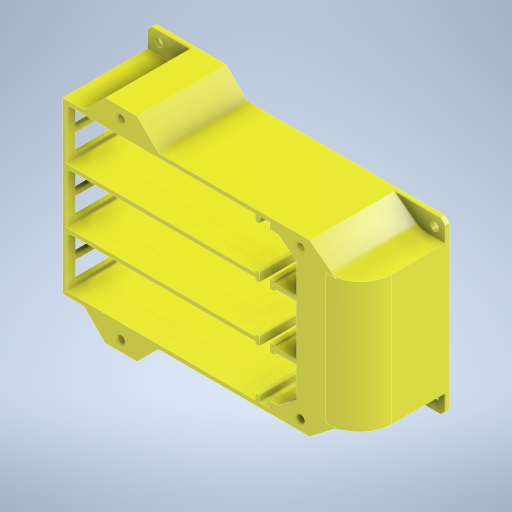
# Autodesk Inventor part: MainBody
Saved by Autodesk Inventor 2024.2 (Build 282272000, 272)
## iProperties
Created: 2024-05-26
Part Number: MainBody
Material: PBT Plastic
Document SubType Name: Modeling
Designer: simon
Density: 1.31 g/cm^3
Appearance: Yellow
Author: simon
Autodesk Inventor part; units mm, degrees
ref_plane "YZ Plane" through (0, 0, 0) normal (1, 0, 0) x (0, 1, 0)
ref_plane "XZ Plane" through (0, 0, 0) normal (0, 1, 0) x (-1, 0, 0)
ref_plane "XY Plane" through (0, 0, 0) normal (0, 0, 1) x (1, 0, 0)
sketch "Sketch1" plane through (0, 0, 0) normal (0, 0, 1) x (1, 0, 0)
  line L0 (0, 0) -> (140, 0)
  line L1 (140, 0) -> (140, 80)
  line L2 (140, 80) -> (0, 80)
  line L3 (0, 80) -> (0, 0)
  line L4 (109.9, 68.55) -> (138, 68.55)
  line L5 (138, 68.55) -> (138, 11.45)
  line L6 (138, 11.45) -> (109.9, 11.45)
  line L7 (109.9, 11.45) -> (109.9, 68.55)
  dimension "d0" = 140
  dimension "d1" = 80
  dimension "d2" = 28.1
  dimension "d3" = 57.1
  dimension "d4" = 11.45
  dimension "d5" = 2
  constraints: 16 end point, 4 parallel, 2 horizontal, 2 perpendicular
  measures "d0" distance of L2.end L1.end
  measures "d1" distance of L1.end L0.end
  measures "d2" distance of L5.end L6.end
  measures "d3" distance of L4.end L5.end
  measures "d4" distance between parallel lines of L2 L4
  measures "d5" distance between parallel lines of L1 L5
extrude "Extrusion1" add sketch "Sketch1" against normal blind 2
sketch "Sketch2" plane through (0, 0, 0) normal (0, 0, 1) x (1, 0, 0)
  line L0 (109.9, 68.55) -> (109.9, 11.45) projected
  line L1 (109.9, 68.55) -> (94.9, 80)
  line L2 (0, 80) -> (140, 80) projected
  line L3 (138, 68.55) -> (109.9, 68.55) projected
  line L4 (109.9, 68.55) -> (113.1962, 68.55)
  line L5 (113.1962, 68.55) -> (98.1962, 80)
  line L6 (98.1962, 80) -> (94.9, 80)
  line L7 (109.9, 11.45) -> (138, 11.45) projected
  line L8 (109.9, 11.45) -> (94.9, 0)
  line L9 (140, 0) -> (0, 0) projected
  line L10 (98.1962, 0) -> (113.1962, 11.45)
  line L11 (113.1962, 11.45) -> (109.9, 11.45)
  line L12 (94.9, 0) -> (98.1962, 0)
  point P0 (113.1962, 11.45)
  point P1 (135, 80)
  point P2 (135, 0)
  dimension "d8" = 2
  dimension "d9" = 15
  dimension "d10" = 2
  dimension "d11" = 15
  constraints: 16 end point, 4 point on line, 3 parallel, 1 collinear, 1 perpendicular
  measures "d8" distance between parallel lines of L5 L1
  measures "d9" horizontal distance of L1.end L0.start
  measures "d10" distance between parallel lines of L10 L8
  measures "d11" horizontal distance of L8.end L0.end
extrude "Extrusion2" add sketch "Sketch2" along normal blind 40
sketch "Sketch3" plane through (109.9, 68.55, -2) normal (0, -1, 0) x (1, 0, 0)
  line L0 (3.2962, 2) -> (28.1, 2) projected
  line L1 (28.1, 2) -> (30.1, 2)
  line L2 (30.1, 2) -> (30.1, 27)
  line L3 (30.1, 27) -> (28.1, 27)
  line L4 (28.1, 27) -> (28.1, 2)
  line L5 (-15, 42) -> (0, 42) projected
  line L6 (0, 42) -> (14, 42)
  line L7 (14, 42) -> (14, 40)
  line L8 (14, 40) -> (0, 40)
  line L9 (0, 40) -> (0, 42)
  arc A0 (30.1, 27) -> (14, 42) centre (15.1001, 27.0404) ccw
  arc A1 (28.1, 27) -> (14, 40) centre (14.1357, 26.0007) ccw
  point P0 (-109.9, 2)
  dimension "d14" = 2
  dimension "d15" = 25
  dimension "d16" = 14
  dimension "d17" = 2
  dimension "d18" = 15
  dimension "d19" = 14
  constraints: 16 end point, 4 parallel, 4 point on circle, 2 centre point, 2 horizontal, 2 perpendicular
  measures "d14" distance of L3.end L2.end
  measures "d15" distance of L1.end L2.end
  measures "d16" distance of L7.end L8.end
  measures "d17" distance of L6.end L7.end
  measures "d18" radius of A0
  measures "d19" radius of A1
extrude "Extrusion3" add sketch "Sketch3" along normal blind 59.1 and the other way blind 2
sketch "Sketch4" plane through (109.9, 9.45, -2) normal (0, -1, 0) x (1, 0, 0)
  line L0 (0.6761, 42) -> (0.6761, 40) projected
  line L1 (0.6761, 42) -> (0.6761, 2)
  line L2 (30.1, 2) -> (-11.7038, 2) projected
  line L3 (30.1, 2) -> (30.1, 0) projected
  line L4 (0.6761, 2) -> (30.1, 2)
  line L5 (30.1, 27) -> (30.1, 2) projected
  line L6 (30.1, 2) -> (30.1, 27)
  line L7 (14, 42) -> (0.6761, 42) projected
  line L8 (0.6761, 42) -> (14, 42)
  arc A0 (30.1, 27) -> (14, 42) centre (15.1001, 27.0404) ccw projected
  arc A1 (30.1, 27) -> (14, 42) centre (15.1001, 27.0404) ccw
  point P0 (-109.9, 2)
  point P1 (0.6761, 40)
  point P2 (25.1, 2)
  point P3 (25.1, 2)
  constraints: 8 end point, 2 collinear, 2 point on circle, 1 centre point, 1 concentric, 1 perpendicular, 1 point on line, 1 vertical
extrude "Extrusion4" add sketch "Sketch4" against normal blind 2
sketch "Sketch5" plane through (109.9, 70.55, -2) normal (0, 1, 0) x (1, 0, 0)
  line L0 (14, -42) -> (0.6761, -42) projected
  line L1 (0.6761, -2) -> (0.6761, -42) projected
  line L2 (0.6761, -42) -> (0.6761, -2)
  line L3 (30.1, -2) -> (0.6761, -2) projected
  line L4 (0.6761, -2) -> (30.1, -2)
  line L5 (30.1, -27) -> (30.1, -2) projected
  line L6 (30.1, -2) -> (30.1, -27)
  line L7 (0.6761, -42) -> (14, -42)
  arc A0 (14, -42) -> (30.1, -27) centre (15.1001, -27.0404) ccw
  point P0 (-109.9, -2)
  constraints: 8 end point, 3 collinear, 2 point on circle, 1 centre point, 1 perpendicular
extrude "Extrusion5" add sketch "Sketch5" against normal blind 2
sketch "Sketch6" plane through (0, 0, 0) normal (0, 0, 1) x (1, 0, 0)
  line L0 (110.5761, 70.55) -> (98.1962, 80) projected
  line L1 (0, 0) -> (98.1962, 0)
  line L2 (98.1962, 0) -> (98.1962, 80)
  line L3 (98.1962, 80) -> (0, 80)
  line L4 (0, 80) -> (0, 0)
  line L5 (2, 2) -> (96.1962, 2)
  line L6 (96.1962, 2) -> (96.1962, 78)
  line L7 (96.1962, 78) -> (2, 78)
  line L8 (2, 78) -> (2, 2)
  line L9 (96.1962, 78) -> (98.1962, 78)
  line L10 (96.1962, 2) -> (98.1962, 2)
  dimension "d34" = 2
  dimension "d35" = 2
  dimension "d36" = 2
  dimension "d37" = 2
  constraints: 20 end point, 4 parallel, 4 perpendicular, 2 horizontal, 2 point on line
  measures "d34" distance between parallel lines of L8 L4
  measures "d35" distance between parallel lines of L5 L1
  measures "d36" distance between parallel lines of L3 L7
  measures "d37" distance between parallel lines of L6 L2
extrude "Extrusion6" add sketch "Sketch6" along normal blind 40 contours L4 L3 L2 L9 L7 L8 L5 L10 L1
sketch "Sketch7" plane through (0, 0, 0) normal (0, 0, 1) x (1, 0, 0)
  line L0 (-10, 53) -> (150, 53) construction
  line L1 (-7.9797, 27) -> (152.0203, 27) construction
  line L2 (0, 80) -> (0, 0) construction
  line L3 (2, 78) -> (97.5201, 78) construction
  line L4 (97.5201, 2) -> (2, 2) construction
  line L5 (2, 2) -> (2, 78) projected
  line L6 (2, 54) -> (92.52, 54)
  line L7 (92.52, 54) -> (92.52, 52)
  line L8 (92.52, 52) -> (2, 52)
  line L9 (2, 52) -> (2, 54)
  line L10 (2, 28) -> (92.52, 28)
  line L11 (92.52, 28) -> (92.52, 26)
  line L12 (92.52, 26) -> (2, 26)
  line L13 (2, 26) -> (2, 28)
  line L14 (0, 80) -> (140, 80) projected
  line L15 (90.5201, 80) -> (92.5201, 80)
  line L16 (92.5201, 80) -> (92.5201, 75)
  line L17 (92.5201, 75) -> (90.5201, 75)
  line L18 (90.5201, 75) -> (90.5201, 80)
  line L19 (97.5201, 78) -> (2, 78) projected
  line L20 (97.5201, 78) -> (97.5201, 75)
  line L21 (97.5201, 75) -> (101.4502, 75)
  line L22 (109.9, 68.55) -> (97.5201, 78) projected
  line L23 (101.4502, 75) -> (97.5201, 78)
  line L24 (97.5201, 78) -> (97.5201, 78)
  line L25 (97.5201, 2) -> (109.9, 11.45) projected
  line L26 (92.5201, 2) -> (90.5201, 2)
  line L27 (90.5201, 2) -> (90.5201, 5)
  line L28 (90.5201, 5) -> (92.5201, 5)
  line L29 (92.5201, 5) -> (92.5201, 2)
  line L30 (92.5201, 55) -> (90.5201, 55)
  line L31 (90.5201, 55) -> (90.5201, 51)
  line L32 (90.5201, 51) -> (92.5201, 51)
  line L33 (92.5201, 51) -> (92.5201, 55)
  line L34 (92.5201, 29) -> (90.52, 29)
  line L35 (90.52, 29) -> (90.52, 25)
  line L36 (90.52, 25) -> (92.5201, 25)
  line L37 (92.5201, 25) -> (92.5201, 29)
  line L38 (97.5201, 55) -> (99.5201, 55)
  line L39 (99.5201, 55) -> (99.5201, 51)
  line L40 (99.5201, 51) -> (97.5201, 51)
  line L41 (97.5201, 51) -> (97.5201, 55)
  line L42 (97.5201, 29) -> (99.5201, 29)
  line L43 (99.5201, 29) -> (99.5201, 25)
  line L44 (99.5201, 25) -> (97.5201, 25)
  line L45 (97.5201, 25) -> (97.5201, 29)
  line L46 (109.9, 68.55) -> (109.9, 11.45) projected
  line L47 (97.5201, 54) -> (109.9, 54)
  line L48 (109.9, 54) -> (109.9, 52)
  line L49 (109.9, 52) -> (97.5201, 52)
  line L50 (97.5201, 52) -> (97.5201, 54)
  line L51 (109.9, 28) -> (97.5201, 28)
  line L52 (97.5201, 28) -> (97.5201, 26)
  line L53 (97.5201, 26) -> (109.9, 26)
  line L54 (109.9, 26) -> (109.9, 28)
  line L55 (97.5201, 2) -> (97.5201, 5)
  line L56 (97.5201, 5) -> (101.4502, 5)
  line L57 (97.5201, 2) -> (101.4502, 5)
  line L58 (0, 0) -> (98.1962, 0) projected
  point P0 (135, 80)
  point P1 (102.7603, 6)
  point P2 (92.5201, 3.5)
  point P3 (91.5201, 55)
  point P4 (90.52, 26)
  point P5 (90.52, 28)
  point P6 (2, 26)
  point P7 (90.5201, 54)
  point P8 (2, 52)
  point P9 (90.5201, 52)
  point P10 (99.5201, 26)
  point P11 (99.5201, 28)
  point P12 (99.5201, 52)
  point P13 (99.5201, 54)
  dimension "d40" = 160
  dimension "d41" = 10
  dimension "d44" = 90.52
  dimension "d45" = 1
  dimension "d46" = 2
  dimension "d47" = 1
  dimension "d48" = 2
  dimension "d49" = 2
  dimension "d54" = 5
  dimension "d55" = 3
  dimension "d56" = 5
  dimension "d57" = 3
  dimension "d60" = 2
  dimension "d61" = 3
  dimension "d62" = 2
  dimension "d63" = 4
  dimension "d64" = 2
  dimension "d65" = 1.9999
  dimension "d66" = 4
  dimension "d67" = 2
  dimension "d68" = 2
  dimension "d69" = 2.0001
  dimension "d70" = 2
  dimension "d71" = 5
  dimension "d72" = 4
  dimension "d73" = 2
  dimension "d74" = 4
  dimension "d75" = 5
  dimension "d78" = 2
  dimension "d79" = 2
  dimension "d80" = 3
  dimension "d81" = 5
  dimension "d105" = 27
  dimension "d106" = 27
  constraints: 98 end point, 20 parallel, 14 perpendicular, 13 point on line, 12 horizontal, 5 collinear, 2 midpoint, 1 vertical
  measures "d40" distance of L0.start L0.end
  measures "d41" distance from line of L0.start L2
  measures "d44" distance of L7.end L8.end
  measures "d45" distance between parallel lines of L6 L0
  measures "d46" distance of L6.end L7.end
  measures "d47" distance between parallel lines of L10 L1
  measures "d48" distance of L10.end L11.end
  measures "d49" distance of L16.end L17.end
  measures "d54" distance between parallel lines of L16 L20
  measures "d55" distance between parallel lines of L3 L21
  measures "d56" distance from line of L3.end L16
  measures "d57" distance between parallel lines of L3 L17
  measures "d60" distance of L27.end L28.end
  measures "d61" distance from line of L26.end L28
  measures "d62" distance of L30.start L30.end
  measures "d63" distance of L32.end L30.start
  measures "d64" distance from line of L0 point (91.52, 55)
  measures "d65" distance from line of L7.end L31
  measures "d66" distance of L36.end L34.start
  measures "d67" distance between parallel lines of L1 L36
  measures "d68" distance from line of L10.end L35
  measures "d69" distance between parallel lines of L37 L35
  measures "d70" distance of L38.start L38.end
  measures "d71" distance between parallel lines of L33 L41
  measures "d72" distance of L38.end L39.end
  measures "d73" distance of L42.start L42.end
  measures "d74" distance of L42.end L43.end
  measures "d75" distance between parallel lines of L37 L45
  measures "d78" distance between parallel lines of L49 L47
  measures "d79" distance of L53.end L51.start
  measures "d80" distance of L4.start L55.end
  measures "d81" distance between parallel lines of L29 L55
  measures "d105" distance between parallel lines of L0 L14
  measures "d106" distance between parallel lines of L1 L58
extrude "Extrusion7" add sketch "Sketch7" along normal blind 40
sketch "Sketch8" plane through (0, 0, -2) normal (-1, 0, 0) x (0, 0, 1)
  line L0 (-10, 66) -> (50, 66) construction
  line L1 (-9.3981, 40) -> (50.6019, 40) construction
  line L2 (-9.3981, 14) -> (50.6019, 14) construction
  line L3 (0, 0) -> (0, 80) construction
  line L4 (0, 80) -> (42, 80) construction
  line L5 (4, 76) -> (38, 76)
  line L6 (38, 76) -> (38, 56)
  line L7 (38, 56) -> (4, 56)
  line L8 (4, 56) -> (4, 76)
  line L9 (42, 0) -> (0, 0) projected
  line L10 (4, 50) -> (38, 50)
  line L11 (38, 50) -> (38, 30)
  line L12 (38, 30) -> (4, 30)
  line L13 (4, 30) -> (4, 50)
  line L14 (4, 24) -> (38, 24)
  line L15 (38, 24) -> (38, 4)
  line L16 (38, 4) -> (4, 4)
  line L17 (4, 4) -> (4, 24)
  line L18 (42, 80) -> (42, 0) projected
  line L19 (38, 67) -> (4, 67)
  line L20 (4, 67) -> (4, 65)
  line L21 (4, 65) -> (38, 65)
  line L22 (38, 65) -> (38, 67)
  line L23 (38, 41) -> (4, 41)
  line L24 (4, 41) -> (4, 39)
  line L25 (4, 39) -> (38, 39)
  line L26 (38, 39) -> (38, 41)
  line L27 (38, 15) -> (4, 15)
  line L28 (4, 15) -> (4, 13)
  line L29 (4, 13) -> (38, 13)
  line L30 (38, 13) -> (38, 15)
  point P0 (2, 0)
  point P1 (4, 15)
  point P2 (38, 39)
  point P3 (4, 41)
  point P4 (4, 67)
  dimension "d82" = 60
  dimension "d83" = 10
  dimension "d87" = 20
  dimension "d88" = 10
  dimension "d89" = 34
  dimension "d90" = 4
  dimension "d91" = 40
  dimension "d93" = 34
  dimension "d94" = 20
  dimension "d95" = 4
  dimension "d96" = 10
  dimension "d97" = 20
  dimension "d98" = 10
  dimension "d99" = 34
  dimension "d100" = 4
  dimension "d103" = 26
  dimension "d104" = 26
  dimension "d107" = 2
  dimension "d108" = 1
  dimension "d109" = 2
  dimension "d110" = 1
  dimension "d111" = 2
  dimension "d112" = 1
  constraints: 54 end point, 12 parallel, 9 horizontal, 6 perpendicular, 6 point on line
  measures "d82" distance of L0.start L0.end
  measures "d83" distance from line of L3 L0.start
  measures "d87" distance of L5.end L6.end
  measures "d88" distance between parallel lines of L0 L7
  measures "d89" distance between parallel lines of L6 L8
  measures "d90" distance between parallel lines of L3 L8
  measures "d91" distance between parallel lines of L1 L4
  measures "d93" distance of L10.start L10.end
  measures "d94" distance of L12.end L10.start
  measures "d95" distance between parallel lines of L3 L13
  measures "d96" distance between parallel lines of L1 L10
  measures "d97" distance of L14.end L15.end
  measures "d98" distance between parallel lines of L14 L2
  measures "d99" distance between parallel lines of L15 L17
  measures "d100" distance between parallel lines of L18 L15
  measures "d103" distance between parallel lines of L1 L2
  measures "d104" distance between parallel lines of L0 L1
  measures "d107" distance between parallel lines of L21 L19
  measures "d108" distance between parallel lines of L0 L21
  measures "d109" distance between parallel lines of L25 L23
  measures "d110" distance between parallel lines of L1 L25
  measures "d111" distance between parallel lines of L29 L27
  measures "d112" distance between parallel lines of L2 L29
extrude "Extrusion8" cut sketch "Sketch8" against normal blind 5 contours L5 L6 L19 L8 | L21 L6 L7 L8 | L10 L11 L23 L13 | L25 L11 L12 L13 | L14 L15 L27 L17 | L29 L15 L16 L17
sketch "Sketch9" plane through (0, 0, -2) normal (0, 0, -1) x (-1, 0, 0)
  line L0 (-140, 0) -> (0, 0) projected
  line L1 (0, 0) -> (-45, 0)
  line L2 (-45, 0) -> (-45, -10)
  line L3 (-45, -10) -> (0, -10)
  line L4 (0, -10) -> (0, 0)
  line L5 (-2, -10) -> (0, -8)
  line L6 (0, 80) -> (0, 0) projected
  line L7 (0, 80) -> (-45, 80)
  line L8 (-45, 80) -> (-45, 90)
  line L9 (-45, 90) -> (0, 90)
  line L10 (0, 90) -> (0, 80)
  line L11 (0, 88) -> (-2, 90)
  line L12 (-45, 0) -> (-35, -10)
  line L13 (-45, 80) -> (-35, 90)
  point P0 (-135, 0)
  point P1 (0, -5)
  point P2 (-45, 85)
  point P3 (0, 85)
  dimension "d113" = 10
  dimension "d114" = 45
  dimension "d115" = 2
  dimension "d116" = 2
  dimension "d117" = 10
  dimension "d118" = 45
  dimension "d119" = 2
  dimension "d120" = 2
  dimension "d121" = 10
  dimension "d122" = 10
  constraints: 24 end point, 6 point on line, 4 parallel, 3 midpoint, 2 horizontal, 2 perpendicular
  measures "d113" distance between parallel lines of L0 L3
  measures "d114" distance from line of L2 point (0, -5)
  measures "d115" distance from line of L4 L5.start
  measures "d116" distance from line of L3 L5.end
  measures "d117" distance between parallel lines of L9 L7
  measures "d118" distance of point (-45, 85) point (0, 85)
  measures "d119" distance from line of L10 L11.end
  measures "d120" distance of L9.end L11.start
  measures "d121" distance from line of L2 L12.end
  measures "d122" distance from line of L13.end L8
extrude "Extrusion9" add sketch "Sketch9" against normal blind 2 contours L0 L4 L5 L3 L12 | L7 L13 L9 L11 L10
chamfer "Chamfer1" distance 2 angle 45 2 edges at (140, 80, -1) (140, 0, -1)
sketch "Sketch10" plane through (0, 0, 0) normal (0, 0, 1) x (1, 0, 0)
  line L0 (45, 80) -> (35, 90) projected
  line L1 (45, 80) -> (35, 90)
  line L2 (35, 90) -> (20, 90)
  line L3 (35, 90) -> (2, 90) projected
  line L4 (20, 90) -> (10, 80)
  line L5 (98.1962, 80) -> (0, 80) projected
  line L6 (10, 80) -> (45, 80)
  line L7 (45, 0) -> (35, -10) projected
  line L8 (45, 0) -> (35, -10)
  line L9 (35, -10) -> (20, -10)
  line L10 (2, -10) -> (35, -10) projected
  line L11 (20, -10) -> (10, 0)
  line L12 (0, 0) -> (45, 0) projected
  line L13 (10, 0) -> (45, 0)
  line L14 (110.5761, 9.45) -> (98.1962, 0)
  line L15 (138, 0) -> (45, 0) projected
  line L16 (110.5761, 9.45) -> (128.5761, 9.45)
  line L17 (140, 9.45) -> (110.5761, 9.45) projected
  line L18 (128.5761, 9.45) -> (116.1962, 0)
  line L19 (116.1962, 0) -> (98.1962, 0)
  line L20 (110.5761, 9.45) -> (98.1962, 0) projected
  line L21 (98.1962, 80) -> (110.5761, 70.55)
  line L22 (110.5761, 70.55) -> (128.5761, 70.55)
  line L23 (138, 68.55) -> (109.9, 68.55) projected
  line L24 (128.5761, 70.55) -> (116.1962, 80)
  line L25 (45, 80) -> (138, 80) projected
  line L26 (98.1962, 80) -> (116.1962, 80)
  line L27 (98.1962, 80) -> (110.5761, 70.55) projected
  point P0 (116.1962, 0)
  dimension "d128" = 10
  dimension "d129" = 25
  dimension "d130" = 10
  dimension "d131" = 25
  dimension "d132" = 18
  dimension "d133" = 18
  constraints: 32 end point, 7 point on line, 6 parallel, 3 collinear
  measures "d128" horizontal distance of L4.end L2.end
  measures "d129" horizontal distance of L0.end L4.end
  measures "d130" horizontal distance of L9.end L11.end
  measures "d131" horizontal distance of L7.end L11.end
  measures "d132" distance of L18.end L14.end
  measures "d133" distance of L24.end L5.start
extrude "Extrusion10" add sketch "Sketch10" along normal blind 40
sketch "Sketch11" plane through (0, 0, 0) normal (0, 0, 1) x (1, 0, 0)
  circle A0 centre (5, 85) radius 2
  circle A1 centre (5, -5) radius 2
  circle A2 centre (135, 75) radius 2
  circle A3 centre (135, 5) radius 2
  line L0 (0, 88) -> (0, 80) projected
  line L1 (20, 90) -> (2, 90) projected
  line L2 (0, 0) -> (0, -8) projected
  line L3 (2, -10) -> (20, -10) projected
  line L4 (140, 2) -> (140, 9.45) projected
  line L5 (116.1962, 0) -> (138, 0) projected
  line L6 (138, 80) -> (116.1962, 80) projected
  line L7 (140, 70.55) -> (140, 78) projected
  dimension "d136" = 4
  dimension "d137" = 4
  dimension "d138" = 4
  dimension "d139" = 4
  dimension "d140" = 5
  dimension "d141" = 5
  dimension "d142" = 5
  dimension "d143" = 5
  dimension "d144" = 5
  dimension "d145" = 5
  dimension "d146" = 5
  dimension "d147" = 5
  constraints: 4 centre point
  measures "d136" diameter of A0
  measures "d137" diameter of A1
  measures "d138" diameter of A2
  measures "d139" diameter of A3
  measures "d140" distance from line of A0.centre L0
  measures "d141" distance from line of A0.centre L1
  measures "d142" distance from line of A1.centre L2
  measures "d143" distance from line of L3 A1.centre
  measures "d144" distance from line of L4 A3.centre
  measures "d145" distance from line of L5 A3.centre
  measures "d146" distance from line of L6 A2.centre
  measures "d147" distance from line of L7 A2.centre
extrude "Extrusion11" cut sketch "Sketch11" against normal blind 4
sketch "Sketch12" plane through (0, 0, 40) normal (0, 0, 1) x (1, 0, 0)
  circle A0 centre (27.5, 85) radius 1.95
  circle A1 centre (27.5, -5) radius 1.95
  circle A2 centre (112, 75) radius 1.95
  circle A3 centre (112, 5) radius 1.95
  line L0 (35, 90) -> (20, 90) projected
  line L1 (20, -10) -> (35, -10) projected
  line L2 (116.1962, 80) -> (45, 80) projected
  line L3 (45, 0) -> (116.1962, 0) projected
  point P0 (0, 0)
  dimension "d150" = 3.9
  dimension "d151" = 3.9
  dimension "d152" = 3.9
  dimension "d153" = 3.9
  dimension "d154" = 5
  dimension "d155" = 7.5
  dimension "d156" = 5
  dimension "d157" = 7.5
  dimension "d158" = 5
  dimension "d159" = 5
  dimension "d160" = 77
  dimension "d161" = 77
  constraints: 4 centre point
  measures "d150" diameter of A0
  measures "d151" diameter of A1
  measures "d152" diameter of A2
  measures "d153" diameter of A3
  measures "d154" distance from line of L0 A0.centre
  measures "d155" horizontal distance of A0.centre L0.start
  measures "d156" distance from line of L1 A1.centre
  measures "d157" horizontal distance of L1.end A1.centre
  measures "d158" distance from line of L2 A2.centre
  measures "d159" distance from line of L3 A3.centre
  measures "d160" horizontal distance of L0.start A2.centre
  measures "d161" horizontal distance of A3.centre L1.end
extrude "Extrusion12" cut sketch "Sketch12" against normal blind 10
fillet "Fillet1" radius 10 2 edges at (128.5761, 9.45, 19.8039) (128.5761, 70.55, 19.8039)
body "Solid1"
